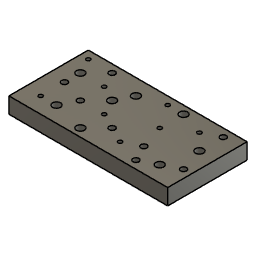
Qatest-Cycle Subprograms (Autodesk Fusion 360 design; units mm, degrees)
Autodesk Fusion 360 part; units mm, degrees
sketch "Sketch1" plane through (0, 0, 0) normal (0, 1, 0) x (1, 0, 0)
  line L0 (-127, -63.5) -> (127, -63.5)
  line L1 (127, -63.5) -> (127, 63.5)
  line L2 (127, 63.5) -> (-127, 63.5)
  line L3 (-127, 63.5) -> (-127, -63.5)
  circle A0 centre (-101.6, -38.1) radius 3.175
  circle A1 centre (-114.3, 50.8) radius 3.175
  circle A2 centre (-63.5, 25.4) radius 3.175
  circle A3 centre (-25.4, -12.7) radius 3.175
  circle A4 centre (25.4, -38.1) radius 3.175
  circle A5 centre (38.1, 12.7) radius 3.175
  circle A6 centre (12.7, 50.8) radius 3.175
  circle A7 centre (76.2, 38.1) radius 3.175
  circle A8 centre (88.9, -38.1) radius 6.35
  circle A9 centre (101.6, 12.7) radius 6.35
  circle A10 centre (-25.4, 38.1) radius 6.35
  circle A11 centre (-38.1, 12.7) radius 6.35
  circle A12 centre (-76.2, -38.1) radius 6.35
  circle A13 centre (-101.6, 25.4) radius 6.35
  circle A14 centre (-25.4, -50.8) radius 6.35
  circle A15 centre (38.1, 50.8) radius 6.35
  circle A16 centre (50.8, -25.4) radius 4.7625
  circle A17 centre (-63.5, -12.7) radius 4.7625
  circle A18 centre (-101.6, 0) radius 4.7625
  circle A19 centre (-76.2, 50.8) radius 4.7625
  circle A20 centre (101.6, 50.8) radius 4.7625
  circle A21 centre (114.3, -25.4) radius 4.7625
  circle A22 centre (63.5, -50.8) radius 4.7625
  circle A23 centre (0, -25.4) radius 4.7625
  dimension "d1" = 6.35
  dimension "d2" = 6.35
  dimension "d3" = 6.35
  dimension "d4" = 6.35
  dimension "d5" = 12.7
  dimension "d6" = 12.7
  dimension "d7" = 9.525
  dimension "d8" = 9.525
  constraint horizontal L0
  constraint vertical L1
  constraint horizontal L2
  constraint vertical L3
  measures "d1" diameter of A0
  measures "d2" diameter of A2
  measures "d3" diameter of A4
  measures "d4" diameter of A7
  measures "d5" diameter of A8
  measures "d6" diameter of A9
  measures "d7" diameter of A18
  measures "d8" diameter of A23
extrude "Extrude1" add sketch "Sketch1" along normal blind 25.4
